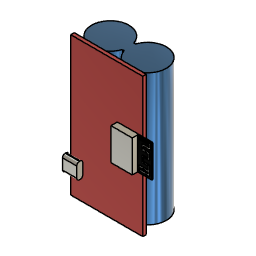
Gnome C3V1 v1 (Autodesk Fusion 360 design; units mm, degrees)
Autodesk Fusion 360 part; units mm, degrees
sketch "Sketch1" plane through (0, 0, 0) normal (0, 0, 1) x (1, 0, 0)
  line L0 (-9.75, -10.5) -> (30.75, -10.5)
  line L1 (30.75, -10.5) -> (30.75, -12.5)
  line L2 (30.75, -12.5) -> (-9.75, -12.5)
  line L3 (-9.75, -12.5) -> (-9.75, -10.5)
  line L4 (21, 0) -> (0, 0) construction
  line L5 (10.5, -10.5) -> (10.5, 0) construction
  line L6 (10, 3.2016) -> (11, 3.2016)
  line L7 (10, -3.2016) -> (11, -3.2016)
  arc A0 (10, 3.2016) -> (10, -3.2016) centre (0, 0) ccw
  arc A1 (10, -3.2016) -> (10.5, 0) centre (0, 0) ccw construction
  arc A2 (11, -3.2016) -> (11, 3.2016) centre (21, 0) ccw
  arc A3 (10.5, 0) -> (11, -3.2016) centre (21, 0) ccw construction
  arc A4 (10.5, 0) -> (10, 3.2016) centre (0, 0) ccw construction
  arc A5 (11, 3.2016) -> (10.5, 0) centre (21, 0) ccw construction
  dimension "d1" = 21
  dimension "d2" = 2
  dimension "d3" = 40.5
  dimension "d9" = 1
  constraint coincident L4.end A0.centre
  constraint equal A0 A2
  constraint horizontal L0
  constraint vertical L1
  constraint horizontal L2
  constraint vertical L3
  constraint coincident L4.start A2.centre
  constraint horizontal L4
  constraint midpoint L0 L5.start
  constraint coincident L4 L5.end
  constraint midpoint L4 L5.end
  constraint tangent L5 A0
  constraint vertical L5
  constraint tangent L0 A0
  constraint horizontal L6
  constraint perpendicular L5 L7
  constraint concentric A0 A1
  constraint concentric A2 A3
  constraint concentric A0 A4
  constraint concentric A2 A5
  constraint equal L6 L7
  measures "d1" diameter of A0
  measures "d2" distance of L0.start L2.end
  measures "d3" distance of L0.start L0.end
  measures "d9" distance of L7.start L7.end
extrude "Extrude1" add sketch "Sketch1" along normal blind 78 contours L0 L1 L2 L3 makes body 1
extrude "Extrude2" add sketch "Sketch1" along normal blind 74 from surface at 2 separate body contours L6 L7 A0 A2 makes body 2
sketch "Sketch4" plane through (0, -12.5, 0) normal (0, -1, 0) x (1, 0, 0)
  line L0 (-9.75, 0) -> (30.75, 0)
  line L1 (30.75, 0) -> (30.75, 78) construction
  line L2 (30.75, 78) -> (-9.75, 78)
  line L3 (-9.75, 78) -> (-9.75, 0) construction
  line L4 (-10.95, 20.7) -> (-2.95, 20.7)
  line L5 (-2.95, 20.7) -> (-2.95, 11.7)
  line L6 (-2.95, 11.7) -> (-10.95, 11.7)
  line L7 (-10.95, 11.7) -> (-10.95, 20.7)
  line L8 (16.45, 48.6368) -> (36.45, 48.6368)
  line L9 (36.45, 48.6368) -> (36.45, 30.6368)
  line L10 (36.45, 30.6368) -> (16.45, 30.6368)
  line L11 (16.45, 30.6368) -> (16.45, 48.6368)
  line L12 (28.45, 48.6368) -> (28.45, 30.6368)
  dimension "d25" = 9
  dimension "d26" = 8
  dimension "d27" = 1.2
  dimension "d28" = 11.7
  dimension "d29" = 18
  dimension "d30" = 20
  dimension "d31" = 12
  dimension "d32" = 5.7
  constraint horizontal L4
  constraint vertical L5
  constraint horizontal L6
  constraint vertical L7
  constraint horizontal L8
  constraint vertical L9
  constraint horizontal L10
  constraint vertical L11
  constraint coincident L8 L12.start
  constraint coincident L10 L12.end
  constraint perpendicular L10 L12
  measures "d25" distance of L4.end L5.end
  measures "d26" distance of L4.start L4.end
  measures "d27" distance of L3 L7
  measures "d28" distance of L0 L6
  measures "d29" distance of L8.end L9.end
  measures "d30" distance of L8.start L8.end
  measures "d31" distance of L11 L12
  measures "d32" distance of L1 L9
extrude "Extrude5" add sketch "Sketch4" along normal blind 3.4 separate body contours L4 L5 L6 L7 makes body 3
extrude "Extrude6" add sketch "Sketch4" along normal blind 0.6 separate body contours L8 L9 L10 L12 makes body 4
extrude "Extrude7" add sketch "Sketch4" along normal blind 3.6 contours L8 L10 L11 L12 bodies 4
fillet "Fillet1" radius 1.5 4 edges at (-6.95, -15.9, 11.7) (-6.95, -12.5, 11.7) (-6.95, -15.9, 20.7) (-6.95, -12.5, 20.7) on bodies 3
sketch "Sketch5" plane through (0, -13.1, 0) normal (0, -1, 0) x (1, 0, 0)
  line L0 (36.45, 48.6368) -> (28.45, 48.6368)
  line L1 (28.45, 48.6368) -> (28.45, 30.6368)
  line L2 (28.45, 30.6368) -> (36.45, 30.6368)
  line L3 (36.45, 30.6368) -> (36.45, 48.6368)
  line L4 (29.3453, 31.8332) -> (35.355, 31.8332)
  line L5 (35.355, 31.8332) -> (35.355, 37.4243)
  line L6 (35.355, 37.4243) -> (31.8287, 37.4243)
  line L7 (31.8287, 37.4243) -> (31.8287, 39.6348)
  line L8 (31.8287, 39.6348) -> (35.3949, 39.6348)
  line L9 (29.3453, 31.8332) -> (29.3453, 32.7601)
  line L10 (29.3453, 32.7601) -> (34.5178, 32.7601)
  line L11 (34.5178, 32.7601) -> (34.5178, 33.6869)
  line L12 (34.5178, 33.6869) -> (29.3453, 33.6869)
  line L13 (29.3453, 33.6869) -> (29.3453, 34.5839)
  line L14 (29.3453, 34.5839) -> (34.5178, 34.5839)
  line L15 (34.5178, 34.5839) -> (34.5178, 36.617)
  line L16 (34.5178, 36.617) -> (31.1393, 36.617)
  line L17 (31.1393, 36.617) -> (31.1393, 40.3179)
  line L18 (31.1393, 40.3179) -> (34.5178, 40.3179)
  line L19 (34.5178, 40.3179) -> (34.5178, 42.5026)
  line L20 (34.5178, 42.5026) -> (31.1393, 42.5026)
  line L21 (31.1393, 42.5026) -> (31.1393, 45.8761)
  line L22 (31.1393, 45.8761) -> (35.8932, 45.8761)
  line L23 (35.8932, 45.8761) -> (35.8932, 44.9244)
  line L24 (35.8932, 44.9244) -> (31.9465, 44.9244)
  line L25 (31.9465, 44.9244) -> (31.9465, 43.4239)
  line L26 (31.9465, 43.4239) -> (35.3949, 43.4239)
  line L27 (35.3949, 43.4239) -> (35.3949, 39.6348)
  line L28 (29.2875, 47.8951) -> (29.2875, 47.1254)
  line L29 (29.2875, 47.1254) -> (35.0233, 47.1254)
  line L30 (35.0233, 47.1254) -> (35.0233, 45.8761)
  line L31 (35.8932, 45.8761) -> (35.8932, 47.8951)
  line L32 (35.8932, 47.8951) -> (29.2875, 47.8951)
  constraint horizontal L4
  constraint perpendicular L4 L5
  constraint perpendicular L5 L6
  constraint perpendicular L6 L7
  constraint perpendicular L5 L8
  constraint perpendicular L4 L9
  constraint perpendicular L9 L10
  constraint perpendicular L10 L11
  constraint perpendicular L11 L12
  constraint perpendicular L12 L13
  constraint perpendicular L13 L14
  constraint perpendicular L14 L15
  constraint perpendicular L13 L16
  constraint perpendicular L16 L17
  constraint perpendicular L17 L18
  constraint perpendicular L18 L19
  constraint perpendicular L19 L20
  constraint perpendicular L20 L21
  constraint perpendicular L21 L22
  constraint perpendicular L20 L23
  constraint perpendicular L23 L24
  constraint perpendicular L24 L25
  constraint perpendicular L25 L26
  constraint vertical L27
  constraint perpendicular L0 L28
  constraint perpendicular L28 L29
  constraint coincident L22 L30.end
  constraint perpendicular L22 L30
  constraint perpendicular L22 L31
  constraint perpendicular L28 L32
extrude "Extrude8" add sketch "Sketch5" along normal blind 0.2 contours L4 L5 L6 L7 L8 L9 L10 L11 L12 L13 L14 L15 L16 L17 L18 L19 L20 L21 L22 L23 L24 L25 L26 L27 | L22 L28 L29 L30 L31 L32 bodies 4
named bodies: "PCB", "Batteries"
